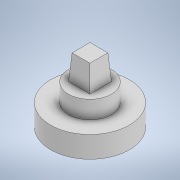
# Autodesk Inventor part: Driveshaft coupling end
Saved by Autodesk Inventor 2021 (Build 250183000, 183)
## iProperties
Created: 2020-03-11
Part Number: Driveshaft coupling end
Material: Generic
Document SubType Name: Modeling
Designer: jstr255
Density: 1 g/cm^3
Appearance: Default
Author: jstr255
Autodesk Inventor part; units mm, degrees
ref_plane "YZ Plane" through (0, 0, 0) normal (1, 0, 0) x (0, 1, 0)
ref_plane "XZ Plane" through (0, 0, 0) normal (0, 1, 0) x (-1, 0, 0)
sketch "Sketch1" plane through (0, 0, 0) normal (0, 1, 0) x (-1, 0, 0)
  circle A0 centre (0, 0) radius 11
  dimension "d0" = 22
  constraints: 1 centre point, 1 coincident
  measures "d0" diameter of A0
extrude "Extrusion1" add sketch "Sketch1" along normal blind 6
sketch "Sketch2" plane through (0, 6, 0) normal (0, 1, 0) x (1, 0, 0)
  circle A0 centre (0, 0) radius 6
  dimension "d3" = 12
  constraints: 1 centre point, 1 coincident
  measures "d3" diameter of A0
extrude "Extrusion2" add sketch "Sketch2" along normal blind 5
sketch "Sketch3" plane through (0, 11, 0) normal (0, 1, 0) x (1, 0, 0)
  line L0 (-3, -3) -> (3, -3)
  line L1 (3, -3) -> (3, 3)
  line L2 (3, 3) -> (-3, 3)
  line L3 (-3, 3) -> (-3, -3)
  point P0 (0, 0)
  dimension "d6" = 6
  dimension "d7" = 6
  constraints: 8 end point, 2 parallel, 1 horizontal, 1 perpendicular
  measures "d6" distance of L2.end L1.end
  measures "d7" distance of L1.end L0.end
ref_plane "Work Plane1" through (0, 18, 0) normal (0, 1, 0) x (1, 0, 0)
sketch "Sketch4" plane through (0, 18, 0) normal (0, 1, 0) x (1, 0, 0)
  line L0 (-2.5, -2.5) -> (2.5, -2.5)
  line L1 (2.5, -2.5) -> (2.5, 2.5)
  line L2 (2.5, 2.5) -> (-2.5, 2.5)
  line L3 (-2.5, 2.5) -> (-2.5, -2.5)
  point P0 (0, 0)
  dimension "d9" = 5
  dimension "d10" = 5
  constraints: 8 end point, 2 parallel, 1 horizontal, 1 perpendicular
  measures "d9" distance of L2.end L1.end
  measures "d10" distance of L1.end L0.end
loft "Loft1" add profiles "Sketch3", "Sketch4"
body "Solid1"
